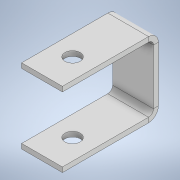
# Autodesk Inventor part: 6x1 BENT
Saved by Autodesk Inventor 2020 (Build 240168000, 168)
## iProperties
Created: 2020-01-01
Part Number: 6x1 BENT
Material: Generic
Document SubType Name: Sheet Metal
Designer: ellio
Density: 1 g/cm^3
Sheet Metal Rule: Default
Appearance: Default
Author: ellio
Autodesk Inventor part; units mm, degrees
ref_plane "YZ Plane" through (0, 0, 0) normal (1, 0, 0) x (0, 1, 0)
ref_plane "XZ Plane" through (0, 0, 0) normal (0, 1, 0) x (-1, 0, 0)
ref_plane "XY Plane" through (0, 0, 0) normal (0, 0, 1) x (1, 0, 0)
sketch "Sketch1" plane through (0, 0, 0) normal (0, 1, 0) x (-1, 0, 0)
  line L0 (0, 0) -> (25.4, 0)
  line L1 (25.4, 0) -> (25.4, -155.575)
  line L2 (25.4, -155.575) -> (0, -155.575)
  line L3 (0, -155.575) -> (0, 0)
  dimension "d0" = 25.4
  dimension "d1" = 155.575
  measures "d0" distance of L1.end L2.end
  measures "d1" distance of L0.end L1.end
extrude "Plate1" add sketch "Sketch1" along normal blind 3.048
sketch "Sketch2" plane through (0, 3.048, 0) normal (0, 1, 0) x (1, 0, 0)
  circle A0 centre (-12.7, 19.05) radius 4.7625
  circle A1 centre (-12.7, 136.525) radius 4.7625
  line L0 (-25.4, 0) -> (-25.4, 155.575) projected
  line L1 (-25.4, 57.15) -> (0, 57.15)
  line L2 (0, 155.575) -> (0, 0) projected
  line L3 (-25.4, 98.425) -> (0, 98.425)
  dimension "d3" = 9.525
  dimension "d4" = 9.525
  constraints: 4 end point, 4 point on line, 2 centre point, 1 horizontal, 1 perpendicular
  measures "d3" diameter of A0
  measures "d4" diameter of A1
hole "Hole1" at (-12.7, 3.048, -19.05) direction (0, -1, 0) diameter 9.525 end through all
sketch "Sketch3" plane through (0, 3.048, 0) normal (0, 1, 0) x (1, 0, 0)
  circle A0 centre (-12.7, 136.525) radius 4.7625
  point P0 (0, 0)
  dimension "d12" = 9.525
  constraints: 1 centre point
  measures "d12" diameter of A0
hole "Hole2" at (-12.7, 3.048, -136.525) direction (0, -1, 0) diameter 9.525 end through all
sketch "Sketch4" plane through (0, 3.048, 0) normal (0, 1, 0) x (1, 0, 0)
  line L0 (-25.4, 0) -> (-25.4, 155.575) projected
  line L1 (-25.4, 57.15) -> (0, 57.15)
  line L2 (-25.4, 98.425) -> (0, 98.425)
  line L3 (0, 155.575) -> (0, 0) projected
  constraints: 4 end point, 3 point on line, 1 horizontal, 1 perpendicular
fold "Fold1" angle 90 bend radius 3.048 thickness 3.048 k factor 0.44 line from (-25.4, 3.048, -57.15) to (0, 3.048, -57.15) line at bend centre moving side (0, 0, -1) folds toward (0, 1, 0)
sketch "Sketch5" plane through (-25.4, 101.0738, -56.7508) normal (0, 0, 1) x (1, 0, 0)
  line L0 (0, -94.9778) -> (0, 0) projected
  line L1 (0, -57.15) -> (25.4, -57.15)
  line L2 (25.4, 0) -> (25.4, -94.9778) projected
  point P0 (25.4, -101.0738)
  constraints: 2 end point, 2 point on line, 1 horizontal
fold "Fold2" angle 90 bend radius 3.048 thickness 3.048 k factor 0.44 line from (-25.4, 43.9238, -56.7508) to (0, 43.9238, -56.7508) line at bend centre moving side (0, 1, 0) folds toward (0, 0, 1)
equation "\"d10\" = Thickness"
equation "\"d18\" = Thickness"
equation "\"d2\" = Thickness"
equation "\"d20\" = BendReliefWidth"
equation "\"d21\" = BendReliefDepth"
equation "\"d22\" = MinimumRemnant"
equation "\"d23\" = TransitionRadius"
equation "\"d25\" = BendRadius"
equation "\"d26\" = BendReliefWidth"
equation "\"d27\" = BendReliefDepth"
equation "\"d28\" = MinimumRemnant"
equation "\"d29\" = TransitionRadius"
equation "\"d31\" = BendRadius"
equation "\"BendRadius\" = Thickness"
equation "\"BendReliefWidth\" = Thickness"
equation "\"BendReliefDepth\" = 0.5 * Thickness"
equation "\"CornerReliefSize\" = 4 * Thickness"
equation "\"MinimumRemnant\" = 2 * Thickness"
equation "\"TransitionRadius\" = BendRadius"
equation "\"JacobiRadiusSize\" = BendRadius"
equation "\"GapSize\" = Thickness"
equation "\"Thickness\" = 3.048"
body "Solid1"
